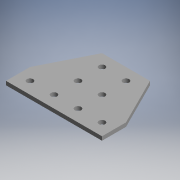
# Autodesk Inventor part: 25-4155
Saved by Autodesk Inventor 2017.3 (Build 213256000, 256)
## iProperties
Part Number: 25-4155
Material: Generic
Catalog Web Link: www.cadenas.de
Description: 25-4155, 25-4155-Black,40-4355, 40-4355-Black, 45-4355, 45-4355-Black-8 Hole Tee Joining Plate
Vendor: 8020
Document SubType Name: Modeling
Designer: partserver
Manufacturer: 8020
Mass: 23.9866 g
Surface Area: 138.789 cm^2
Volume: 23.9866 cm^3
Density: 1 g/cm^3
Appearance: PSOLRGB-191-191-191
Category: PARTsolutions
Company: 8020
Title: 25-4155
Author: Cadenas PARTsolutions
Comments: 8 Hole Tee Joining Plate
PSOL_IDENT_0: {$CADENAS_DATA\23d-libs\8020\metric\joining_plates\25_4155.prj},217 {VTYP=3D},{NB=25-4155},{LINA=25-
PSOL_IDENT_1: 4155},{NN=25-4155, 25-4155-Black,40-4355, 40-4355-Black, 45-4355, 45-4355-Black},{DATE=31.07.2020 09
PSOL_IDENT_2: :21:28},{GEOMDATE=16.01.2019 18:32:00},{VERSION=},{LINEID=10},{WBVAR=},{WBNUMERIC=}  {NB=25-4155},{L
PSOL_IDENT_3: INA=25-4155},{KT=DUMMY},{PN=25-4155},{A=100.00},{B=75.00},{C=50.00},{D=25.00},{E=12.50},{F=25.00},{T=
PSOL_IDENT_4: 4.00},{DIA=6.350},{W=.076},{A1=12.5000},{C1=37.500},{C3=62.500},{C4=87.500},{COLOR=.75,.75,.75}
NB: 25-4155
NN: 25-4155, 25-4155-Black,40-4355, 40-4355-Black, 45-4355, 45-4355-Black
NT: 8 Hole Tee Joining Plate
NBSYN: $PN.
LINA: 25-4155
CATALOG: 80/20
PN: 25-4155
A: 100
B: 75
C: 50
D: 25
E: 12.5
F: 25
T: 4
DIA: 6.35
W: .076
SUPPLIER: 8020
ARTICLENO: 25-4155
BOMINFO: 25-4155
CREATOR: CADENAS GmbH
Autodesk Inventor part; units mm, degrees
ref_plane "YZ Plane" through (0, 0, 0) normal (1, 0, 0) x (0, 1, 0)
ref_plane "XZ Plane" through (0, 0, 0) normal (0, 1, 0) x (-1, 0, 0)
ref_plane "XY Plane" through (0, 0, 0) normal (0, 0, 1) x (1, 0, 0)
sketch "Sketch_1" plane through (0, 0, 0) normal (0, 0, 1) x (1, 0, 0)
  line L0 (-50, 25) -> (-50, 0)
  line L1 (-50, 0) -> (50, 0)
  line L2 (50, 0) -> (50, 25)
  line L3 (50, 25) -> (25, 75)
  line L4 (25, 75) -> (-25, 75)
  line L5 (-25, 75) -> (-50, 25)
  circle A0 centre (37.5, 12.5) radius 3.175
  circle A1 centre (12.5, 12.5) radius 3.175
  circle A2 centre (12.5, 37.5) radius 3.175
  circle A3 centre (12.5, 62.5) radius 3.175
  circle A4 centre (-12.5, 37.5) radius 3.175
  circle A5 centre (-12.5, 12.5) radius 3.175
  circle A6 centre (-12.5, 62.5) radius 3.175
  circle A7 centre (-37.5, 12.5) radius 3.175
  constraints: 12 end point, 8 centre point
extrude "Extrusion1" add sketch "Sketch_1" along normal blind 4
body "Solid1"
